Autodesk Fusion 360 part; units mm, degrees
(part 2 of 2)
  spline S382 degree 3 poles (93.789, 651.4002) (93.7155, 651.4002) (93.7155, 651.4737) (93.642, 651.4737) knots 0 0 0 0 1 1 1 1
  spline S383 degree 3 poles (93.642, 651.4737) (86.5858, 656.8394) (73.8699, 659.3385) (72.5468, 659.559) knots 0 0 0 0 1 1 1 1
  spline S384 degree 3 poles (72.5468, 659.559) (72.4733, 659.559) (72.3998, 659.559) (72.3263, 659.559) knots 0 0 0 0 1 1 1 1
  spline S385 degree 3 poles (72.3263, 659.559) (69.5332, 659.706) (66.7401, 659.7795) (63.947, 659.9265) knots 0 0 0 0 1 1 1 1
  spline S386 degree 3 poles (63.947, 659.9265) (63.5795, 659.9265) (63.212, 660) (62.8445, 660) knots 0 0 0 0 1 1 1 1
  spline S387 degree 3 poles (62.8445, 660) (62.6975, 660) (62.624, 660) (62.477, 660) knots 0 0 0 0 1 1 1 1
  spline S388 degree 3 poles (62.477, 660) (59.8309, 659.4855) (57.1848, 659.0445) (54.5387, 658.53) knots 0 0 0 0 1 1 1 1
  spline S389 degree 3 poles (54.5387, 658.53) (54.3917, 658.4565) (54.1712, 658.3829) (54.0242, 658.3094) knots 0 0 0 0 1 1 1 1
  spline S390 degree 3 poles (54.0242, 658.3094) (53.8772, 658.2359) (53.8037, 658.1624) (53.7302, 658.0889) knots 0 0 0 0 1 1 1 1
  line L13 (53.7302, 658.0889) -> (53.3627, 657.7214)
  spline S391 degree 3 poles (53.3627, 657.7214) (53.2892, 657.6479) (53.2157, 657.5744) (53.0687, 657.5009) knots 0 0 0 0 1 1 1 1
  spline S392 degree 3 poles (53.0687, 657.5009) (52.1867, 657.0599) (51.3781, 656.6924) (50.5696, 656.2514) knots 0 0 0 0 1 1 1 1
  line L14 (50.5696, 656.2514) -> (50.1286, 655.9574)
  spline S393 degree 3 poles (50.1286, 655.9574) (49.9816, 655.8104) (49.8346, 655.6634) (49.6876, 655.4429) knots 0 0 0 0 1 1 1 1
  spline S394 degree 3 poles (49.6876, 655.4429) (49.6141, 655.3694) (49.6141, 655.2223) (49.5406, 655.1488) knots 0 0 0 0 1 1 1 1
  spline S395 degree 3 poles (49.5406, 655.1488) (47.0415, 653.2378) (45.2039, 650.8857) (44.1014, 647.9456) knots 0 0 0 0 1 1 1 1
  spline S396 degree 3 poles (44.1014, 647.9456) (43.9544, 647.5781) (44.0279, 647.1371) (44.2484, 646.7696) knots 0 0 0 0 1 1 1 1
  spline S397 degree 3 poles (44.2484, 646.7696) (44.4689, 646.4021) (44.7629, 645.9611) (44.9834, 645.5935) knots 0 0 0 0 1 1 1 1
  spline S398 degree 3 poles (44.9834, 645.5935) (45.645, 644.7115) (46.3065, 643.8295) (47.0415, 642.874) knots 0 0 0 0 1 1 1 1
  spline S399 degree 3 poles (47.0415, 642.874) (51.6722, 636.1852) (56.2293, 629.3495) (60.9335, 622.7343) knots 0 0 0 0 1 1 1 1
  spline S400 degree 3 poles (60.9335, 622.7343) (62.2565, 620.8968) (62.5505, 618.9122) (62.918, 616.9276) knots 0 0 0 0 1 1 1 1
  spline S401 degree 3 poles (62.918, 616.9276) (63.4325, 613.6935) (63.8735, 610.4594) (64.3146, 607.2253) knots 0 0 0 0 1 1 1 1
  spline S402 degree 3 poles (64.3146, 607.2253) (64.4616, 606.1228) (64.2411, 605.0202) (63.653, 604.0647) knots 0 0 0 0 1 1 1 1
  spline S403 degree 3 poles (63.653, 604.0647) (62.771, 602.5212) (61.8155, 601.0511) (60.7864, 599.5811) knots 0 0 0 0 1 1 1 1
  spline S404 degree 3 poles (60.7864, 599.5811) (60.4189, 599.0666) (59.9044, 598.552) (59.3164, 598.258) knots 0 0 0 0 1 1 1 1
  spline S405 degree 3 poles (59.3164, 598.258) (57.4053, 597.376) (56.5233, 595.7589) (55.8618, 593.9214) knots 0 0 0 0 1 1 1 1
  spline S406 degree 3 poles (55.8618, 593.9214) (55.2738, 592.1573) (54.2447, 590.8343) (52.4072, 590.0258) knots 0 0 0 0 1 1 1 1
  spline S407 degree 3 poles (52.4072, 590.0258) (48.144, 588.0412) (43.8809, 585.9096) (39.6913, 583.7046) knots 0 0 0 0 1 1 1 1
  spline S408 degree 3 poles (39.6913, 583.7046) (36.6042, 582.014) (34.7666, 579.0004) (33.5906, 575.8398) knots 0 0 0 0 1 1 1 1
  spline S409 degree 3 poles (33.5906, 575.8398) (32.341, 572.4587) (31.8265, 568.8571) (30.6505, 565.476) knots 0 0 0 0 1 1 1 1
  spline S410 degree 3 poles (30.6505, 565.476) (30.577, 565.182) (30.43, 564.9615) (30.3565, 564.6674) knots 0 0 0 0 1 1 1 1
  spline S411 degree 3 poles (30.3565, 564.6674) (30.283, 564.4469) (30.283, 564.2999) (30.283, 564.0794) knots 0 0 0 0 1 1 1 1
  spline S412 degree 3 poles (30.283, 564.0794) (30.283, 563.6384) (30.3565, 563.1974) (30.3565, 562.6829) knots 0 0 0 0 1 1 1 1
  spline S413 degree 3 poles (30.3565, 562.6829) (30.3565, 560.3308) (29.9155, 558.1257) (29.0334, 556.1412) knots 0 0 0 0 1 1 1 1
  spline S414 degree 3 poles (29.0334, 556.1412) (28.9599, 556.0677) (28.9599, 555.9207) (28.9599, 555.8472) knots 0 0 0 0 1 1 1 1
  spline S415 degree 3 poles (28.9599, 555.8472) (28.6659, 554.0831) (28.3719, 552.6131) (28.2249, 551.0695) knots 0 0 0 0 1 1 1 1
  spline S416 degree 3 poles (28.2249, 551.0695) (27.7839, 547.6884) (27.6369, 544.3808) (29.842, 541.5142) knots 0 0 0 0 1 1 1 1
  spline S417 degree 3 poles (29.842, 541.5142) (31.2385, 539.6767) (33.0026, 538.1331) (34.3991, 536.3691) knots 0 0 0 0 1 1 1 1
  spline S418 degree 3 poles (34.3991, 536.3691) (34.9871, 535.634) (35.5016, 534.605) (35.4281, 533.723) knots 0 0 0 0 1 1 1 1
  spline S419 degree 3 poles (35.4281, 533.723) (35.3546, 531.8854) (35.2076, 530.1214) (34.9136, 528.2838) knots 0 0 0 0 1 1 1 1
  spline S420 degree 3 poles (34.9136, 528.2838) (34.7666, 527.1078) (33.2966, 526.6667) (32.5616, 527.4753) knots 0 0 0 0 1 1 1 1
  spline S421 degree 3 poles (32.5616, 527.4753) (32.1205, 527.9898) (31.606, 528.4308) (30.871, 528.6513) knots 0 0 0 0 1 1 1 1
  spline S422 degree 3 poles (30.871, 528.6513) (30.283, 528.8718) (29.6215, 528.6513) (29.3274, 528.1368) knots 0 0 0 0 1 1 1 1
  spline S423 degree 3 poles (29.3274, 528.1368) (28.6659, 527.1813) (28.2984, 526.0787) (28.0779, 524.9027) knots 0 0 0 0 1 1 1 1
  spline S424 degree 3 poles (28.0779, 524.9027) (27.8574, 523.9472) (26.6814, 523.5062) (25.8728, 524.0942) knots 0 0 0 0 1 1 1 1
  spline S425 degree 3 poles (25.8728, 524.0942) (25.3583, 524.5352) (24.7703, 524.9027) (24.1088, 525.1967) knots 0 0 0 0 1 1 1 1
  spline S426 degree 3 poles (24.1088, 525.1967) (23.3003, 525.5642) (21.9037, 525.7847) (21.0217, 525.5642) knots 0 0 0 0 1 1 1 1
  spline S427 degree 3 poles (21.0217, 525.5642) (16.0235, 524.3147) (12.0544, 521.4481) (8.3058, 518.067) knots 0 0 0 0 1 1 1 1
  spline S428 degree 3 poles (8.3058, 518.067) (7.7913, 517.626) (7.5708, 516.8174) (7.4972, 516.1559) knots 0 0 0 0 1 1 1 1
  spline S429 degree 3 poles (7.4972, 516.1559) (7.2032, 514.2448) (6.9092, 512.4073) (5.5127, 510.8637) knots 0 0 0 0 1 1 1 1
  spline S430 degree 3 poles (5.5127, 510.8637) (3.8956, 509.0997) (4.1161, 506.9681) (4.0426, 504.763) knots 0 0 0 0 1 1 1 1
  spline S431 degree 3 poles (4.0426, 504.763) (3.9691, 502.4845) (4.1161, 500.4999) (6.3212, 499.1769) knots 0 0 0 0 1 1 1 1
  spline S432 degree 3 poles (6.3212, 499.1769) (6.4682, 499.1034) (6.7622, 498.8094) (6.7622, 498.6623) knots 0 0 0 0 1 1 1 1
  spline S433 degree 3 poles (6.7622, 498.6623) (6.6152, 496.4573) (7.1297, 493.9582) (5.4392, 492.1941) knots 0 0 0 0 1 1 1 1
  spline S434 degree 3 poles (5.4392, 492.1941) (2.9401, 489.548) (1.6906, 486.6815) (1.9846, 483.0799) knots 0 0 0 0 1 1 1 1
  spline S435 degree 3 poles (1.9846, 483.0799) (2.2051, 480.8013) (1.9846, 478.5227) (2.0581, 476.2441) knots 0 0 0 0 1 1 1 1
  spline S436 degree 3 poles (2.0581, 476.2441) (2.0581, 475.3621) (2.7196, 474.1861) (3.4546, 473.598) knots 0 0 0 0 1 1 1 1
  spline S437 degree 3 poles (3.4546, 473.598) (5.5127, 472.0545) (6.0272, 469.6289) (5.9537, 467.4974) knots 0 0 0 0 1 1 1 1
  spline S438 degree 3 poles (5.9537, 467.4974) (5.7332, 462.4992) (4.1161, 457.7216) (2.4256, 452.9439) knots 0 0 0 0 1 1 1 1
  spline S439 degree 3 poles (2.4256, 452.9439) (1.2495, 449.5628) (1.1025, 445.8877) (0.294, 442.3596) knots 0 0 0 0 1 1 1 1
  spline S440 degree 3 poles (0.294, 442.3596) (-0.2205, 440.0075) (0.441, 437.8024) (1.6171, 436.2589) knots 0 0 0 0 1 1 1 1
  spline S441 degree 3 poles (1.6171, 436.2589) (3.3076, 434.1273) (5.6597, 432.2898) (8.5998, 431.9958) knots 0 0 0 0 1 1 1 1
  spline S442 degree 3 poles (8.5998, 431.9958) (9.1878, 431.9222) (9.8493, 432.5838) (10.3638, 433.0248) knots 0 0 0 0 1 1 1 1
  spline S443 degree 3 poles (10.3638, 433.0248) (11.8339, 434.3478) (12.7894, 434.1273) (13.3774, 432.2163) knots 0 0 0 0 1 1 1 1
  spline S444 degree 3 poles (13.3774, 432.2163) (14.48, 428.6881) (14.774, 425.0865) (13.9655, 421.4114) knots 0 0 0 0 1 1 1 1
  spline S445 degree 3 poles (13.9655, 421.4114) (13.6714, 420.0149) (13.7449, 418.4713) (13.5244, 417.0748) knots 0 0 0 0 1 1 1 1
  spline S446 degree 3 poles (13.5244, 417.0748) (13.4509, 416.3397) (13.0834, 415.6047) (12.8629, 414.8697) knots 0 0 0 0 1 1 1 1
  spline S447 degree 3 poles (12.8629, 414.8697) (12.7159, 414.7227) (12.6424, 414.5022) (12.4954, 414.3552) knots 0 0 0 0 1 1 1 1
  spline S448 degree 3 poles (12.4954, 414.3552) (11.3194, 410.533) (9.1143, 407.2989) (6.6887, 404.1383) knots 0 0 0 0 1 1 1 1
  spline S449 degree 3 poles (6.6887, 404.1383) (5.5862, 402.7418) (5.2922, 401.0512) (5.9537, 399.1402) knots 0 0 0 0 1 1 1 1
  spline S450 degree 3 poles (5.9537, 399.1402) (7.6443, 394.3625) (11.6869, 392.3045) (15.803, 390.3199) knots 0 0 0 0 1 1 1 1
  spline S451 degree 3 poles (15.803, 390.3199) (16.685, 389.8789) (17.5671, 389.6584) (18.4491, 389.2909) knots 0 0 0 0 1 1 1 1
  spline S452 degree 3 poles (18.4491, 389.2909) (20.1397, 388.5559) (22.0507, 388.8499) (22.7857, 390.4669) knots 0 0 0 0 1 1 1 1
  spline S453 degree 3 poles (22.7857, 390.4669) (24.6233, 394.5096) (28.3719, 396.4206) (31.3855, 399.1402) knots 0 0 0 0 1 1 1 1
  spline S454 degree 3 poles (31.3855, 399.1402) (32.8556, 400.5367) (34.3991, 401.8598) (35.7957, 403.3298) knots 0 0 0 0 1 1 1 1
  spline S455 degree 3 poles (35.7957, 403.3298) (37.4127, 405.0939) (38.9563, 403.5503) (40.4998, 403.4033) knots 0 0 0 0 1 1 1 1
  spline S456 degree 3 poles (40.4998, 403.4033) (41.6758, 403.3298) (41.4553, 402.2273) (41.6758, 401.4923) knots 0 0 0 0 1 1 1 1
  spline S457 degree 3 poles (41.6758, 401.4923) (43.0724, 397.5967) (40.7203, 394.4361) (39.5443, 391.1284) knots 0 0 0 0 1 1 1 1
  spline S458 degree 3 poles (39.5443, 391.1284) (39.5443, 391.0549) (39.5443, 391.0549) (39.4708, 390.9814) knots 0 0 0 0 1 1 1 1
  spline S459 degree 3 poles (39.4708, 390.9814) (38.9563, 390.0259) (38.5152, 388.9969) (38.0742, 387.9678) knots 0 0 0 0 1 1 1 1
  spline S460 degree 2 poles (38.0742, 387.9678) (38.0742, 387.8943) (38.0007, 387.8943) knots 0 0 0 1 1 1
  spline S461 degree 3 poles (38.0007, 387.8943) (37.6332, 387.1593) (37.1922, 386.4243) (36.8247, 385.6157) knots 0 0 0 0 1 1 1 1
  spline S462 degree 3 poles (36.8247, 385.6157) (36.8982, 385.6157) (37.0452, 385.6157) (37.1187, 385.6157) knots 0 0 0 0 1 1 1 1
  spline S463 degree 3 poles (37.1187, 385.6157) (35.5751, 381.5731) (34.3991, 377.604) (34.0316, 376.0604) knots 0 0 0 0 1 1 1 1
  spline S464 degree 3 poles (34.0316, 376.0604) (33.9581, 375.8399) (33.8846, 375.6194) (33.8111, 375.3254) knots 0 0 0 0 1 1 1 1
  spline S465 degree 3 poles (33.8111, 375.3254) (33.6641, 374.6639) (33.4436, 374.0024) (33.5171, 373.3408) knots 0 0 0 0 1 1 1 1
  spline S466 degree 3 poles (33.5171, 373.3408) (33.5906, 372.6793) (33.8111, 371.8708) (34.3256, 371.5768) knots 0 0 0 0 1 1 1 1
  spline S467 degree 3 poles (34.3256, 371.5768) (35.7957, 370.4743) (37.3392, 369.4452) (39.0298, 368.6367) knots 0 0 0 0 1 1 1 1
  spline S468 degree 3 poles (39.0298, 368.6367) (42.0434, 367.1667) (42.9254, 364.4471) (43.1459, 361.5805) knots 0 0 0 0 1 1 1 1
  spline S469 degree 3 poles (43.1459, 361.5805) (43.3664, 357.8318) (42.9989, 353.9362) (42.9989, 350.1876) knots 0 0 0 0 1 1 1 1
  spline S470 degree 3 poles (42.9989, 350.1876) (42.9989, 349.1586) (43.2929, 348.203) (43.2194, 347.174) knots 0 0 0 0 1 1 1 1
  spline S471 degree 3 poles (43.2194, 347.174) (43.0724, 342.9844) (42.8519, 338.8682) (42.4844, 334.6786) knots 0 0 0 0 1 1 1 1
  spline S472 degree 3 poles (42.4844, 334.6786) (42.4844, 334.2376) (41.6023, 333.5761) (41.0878, 333.4291) knots 0 0 0 0 1 1 1 1
  spline S473 degree 3 poles (41.0878, 333.4291) (40.1323, 333.2086) (39.0298, 333.282) (38.0742, 333.3556) knots 0 0 0 0 1 1 1 1
  spline S474 degree 3 poles (38.0742, 333.3556) (36.8982, 333.4291) (36.3102, 332.988) (35.9427, 331.959) knots 0 0 0 0 1 1 1 1
  spline S475 degree 3 poles (35.9427, 331.959) (34.0316, 326.7403) (33.5906, 321.4482) (35.7221, 316.156) knots 0 0 0 0 1 1 1 1
  spline S476 degree 3 poles (35.7221, 316.156) (35.9427, 315.6415) (35.9427, 314.98) (35.9427, 314.392) knots 0 0 0 0 1 1 1 1
  spline S477 degree 3 poles (35.9427, 314.392) (35.5751, 310.6433) (35.5751, 307.1152) (38.8092, 304.3221) knots 0 0 0 0 1 1 1 1
  spline S478 degree 3 poles (38.8092, 304.3221) (41.2348, 302.2641) (41.8963, 298.0009) (40.0588, 295.4283) knots 0 0 0 0 1 1 1 1
  spline S479 degree 3 poles (40.0588, 295.4283) (39.9118, 295.2078) (39.8383, 294.8403) (39.6178, 294.6933) knots 0 0 0 0 1 1 1 1
  spline S480 degree 3 poles (39.6178, 294.6933) (37.4862, 293.5173) (35.2811, 292.4147) (33.0761, 291.2387) knots 0 0 0 0 1 1 1 1
  spline S481 degree 3 poles (33.0761, 291.2387) (32.9291, 291.0917) (32.8556, 290.9447) (32.7086, 290.8712) knots 0 0 0 0 1 1 1 1
  spline S482 degree 3 poles (32.7086, 290.8712) (30.6505, 289.6216) (28.6659, 288.2251) (26.6079, 287.049) knots 0 0 0 0 1 1 1 1
  spline S483 degree 3 poles (26.6079, 287.049) (24.0353, 285.6525) (21.2422, 284.55) (18.5961, 283.374) knots 0 0 0 0 1 1 1 1
  line L15 (18.5961, 283.374) -> (17.9346, 282.8594)
  spline S484 degree 3 poles (17.9346, 282.8594) (16.097, 280.6544) (14.186, 278.3758) (12.3484, 276.1707) knots 0 0 0 0 1 1 1 1
  spline S485 degree 3 poles (12.3484, 276.1707) (12.1279, 275.8767) (11.8339, 275.5092) (11.4664, 275.4357) knots 0 0 0 0 1 1 1 1
  spline S486 degree 3 poles (11.4664, 275.4357) (8.9673, 274.4802) (8.8203, 272.3486) (8.5998, 270.07) knots 0 0 0 0 1 1 1 1
  spline S487 degree 3 poles (8.5998, 270.07) (8.3058, 267.2034) (8.0118, 264.1899) (7.2032, 261.4703) knots 0 0 0 0 1 1 1 1
  spline S488 degree 3 poles (7.2032, 261.4703) (6.5417, 259.1917) (5.0717, 257.1336) (4.0426, 255.0021) knots 0 0 0 0 1 1 1 1
  spline S489 degree 3 poles (4.0426, 255.0021) (3.6751, 254.267) (3.4546, 253.3115) (3.5281, 252.503) knots 0 0 0 0 1 1 1 1
  spline S490 degree 3 poles (3.5281, 252.503) (3.9691, 247.3578) (6.4682, 243.1682) (9.7758, 239.346) knots 0 0 0 0 1 1 1 1
  spline S491 degree 3 poles (9.7758, 239.346) (11.4664, 237.435) (12.8629, 235.3034) (14.627, 233.4658) knots 0 0 0 0 1 1 1 1
  spline S492 degree 3 poles (14.627, 233.4658) (19.9927, 227.9532) (23.1533, 220.897) (28.4454, 215.3843) knots 0 0 0 0 1 1 1 1
  spline S493 degree 3 poles (28.4454, 215.3843) (29.1069, 214.7227) (29.6215, 213.9142) (30.3565, 213.4732) knots 0 0 0 0 1 1 1 1
  spline S494 degree 3 poles (30.3565, 213.4732) (32.341, 212.1502) (32.9291, 210.1656) (33.2966, 208.034) knots 0 0 0 0 1 1 1 1
  spline S495 degree 3 poles (33.2966, 208.034) (34.0316, 203.5504) (35.3546, 199.2873) (37.6332, 195.3182) knots 0 0 0 0 1 1 1 1
  spline S496 degree 3 poles (37.6332, 195.3182) (40.4263, 190.32) (42.9254, 185.1013) (45.939, 180.2502) knots 0 0 0 0 1 1 1 1
  spline S497 degree 3 poles (45.939, 180.2502) (47.997, 176.9426) (50.6431, 174.076) (53.1422, 171.0624) knots 0 0 0 0 1 1 1 1
  spline S498 degree 3 poles (53.1422, 171.0624) (54.9063, 168.8573) (56.7438, 166.7257) (58.5079, 164.5207) knots 0 0 0 0 1 1 1 1
  spline S499 degree 3 poles (58.5079, 164.5207) (58.8754, 164.0061) (59.1694, 163.1976) (59.0224, 162.6831) knots 0 0 0 0 1 1 1 1
  spline S500 degree 3 poles (59.0224, 162.6831) (58.2139, 158.6405) (58.9489, 154.6713) (59.9044, 150.7757) knots 0 0 0 0 1 1 1 1
  spline S501 degree 3 poles (59.9044, 150.7757) (60.2719, 149.0852) (59.8309, 148.5706) (58.3609, 148.2766) knots 0 0 0 0 1 1 1 1
  spline S502 degree 3 poles (58.3609, 148.2766) (54.5388, 147.3946) (51.3047, 145.0425) (48.5116, 142.5434) knots 0 0 0 0 1 1 1 1
  spline S503 degree 3 poles (48.5116, 142.5434) (46.086, 140.3384) (44.1014, 137.3983) (43.0724, 133.9436) knots 0 0 0 0 1 1 1 1
  spline S504 degree 3 poles (43.0724, 133.9436) (42.1169, 130.489) (41.1613, 127.1079) (41.5288, 123.5063) knots 0 0 0 0 1 1 1 1
  line L16 (41.5288, 123.5063) -> (41.5288, 123.4328)
  spline S505 degree 3 poles (41.5288, 123.4328) (41.5288, 123.1388) (41.5288, 122.9183) (41.5288, 122.6243) knots 0 0 0 0 1 1 1 1
  spline S506 degree 3 poles (41.5288, 122.6243) (41.5288, 122.5508) (41.5288, 122.4038) (41.5288, 122.3303) knots 0 0 0 0 1 1 1 1
  spline S507 degree 3 poles (41.5288, 122.3303) (41.6758, 121.4482) (41.8228, 120.5662) (42.1169, 119.7577) knots 0 0 0 0 1 1 1 1
  spline S508 degree 3 poles (42.1169, 119.7577) (42.7049, 118.4347) (43.4399, 117.1116) (44.1014, 115.7886) knots 0 0 0 0 1 1 1 1
  spline S509 degree 3 poles (44.1014, 115.7886) (44.3219, 115.274) (44.8364, 114.9801) (45.4245, 115.0535) knots 0 0 0 0 1 1 1 1
  spline S510 degree 3 poles (45.4245, 115.0535) (46.674, 115.127) (47.9235, 115.2005) (49.1731, 115.2005) knots 0 0 0 0 1 1 1 1
  spline S511 degree 3 poles (49.1731, 115.2005) (49.9081, 115.2005) (50.6431, 115.0535) (51.3047, 114.7596) knots 0 0 0 0 1 1 1 1
  spline S512 degree 3 poles (51.3047, 114.7596) (56.8908, 112.334) (62.477, 109.8349) (67.4752, 106.3068) knots 0 0 0 0 1 1 1 1
  spline S513 degree 3 poles (67.4752, 106.3068) (67.6222, 106.1598) (67.7692, 106.0128) (67.9162, 105.7923) knots 0 0 0 0 1 1 1 1
  spline S514 degree 3 poles (67.9162, 105.7923) (68.0632, 105.7188) (68.2102, 105.7188) (68.3572, 105.6452) knots 0 0 0 0 1 1 1 1
  spline S515 degree 2 poles (68.3572, 105.6452) (72.3998, 102.1906) (69.6067, 95.9429) knots 0 0 0 1 1 1
  spline S516 degree 3 poles (69.6067, 95.9429) (68.7247, 94.1054) (67.9897, 92.0473) (66.8136, 90.3568) knots 0 0 0 0 1 1 1 1
  spline S517 degree 3 poles (66.8136, 90.3568) (64.3881, 86.9021) (63.506, 83.08) (63.1385, 78.9639) knots 0 0 0 0 1 1 1 1
  spline S518 degree 3 poles (63.1385, 78.9639) (63.065, 78.0084) (63.065, 76.9793) (62.6975, 76.1708) knots 0 0 0 0 1 1 1 1
  spline S519 degree 3 poles (62.6975, 76.1708) (61.154, 73.3042) (61.9625, 70.5847) (62.9915, 67.8651) knots 0 0 0 0 1 1 1 1
  spline S520 degree 3 poles (62.9915, 67.8651) (64.5351, 63.8224) (67.0341, 60.7353) (70.4153, 58.0893) knots 0 0 0 0 1 1 1 1
  spline S521 degree 3 poles (70.4153, 58.0893) (72.2528, 56.6927) (73.5024, 54.5612) (74.9724, 52.7236) knots 0 0 0 0 1 1 1 1
  spline S522 degree 3 poles (74.9724, 52.7236) (76.1484, 51.1801) (77.251, 49.6365) (78.28, 48.0194) knots 0 0 0 0 1 1 1 1
  spline S523 degree 3 poles (78.28, 48.0194) (78.3535, 47.8724) (78.427, 47.7254) (78.5005, 47.5784) knots 0 0 0 0 1 1 1 1
  line L17 (78.5005, 47.5784) -> (80.1911, 46.3289)
  spline S524 degree 3 poles (80.1911, 46.3289) (82.1756, 46.4024) (84.1602, 46.5494) (85.9243, 45.0793) knots 0 0 0 0 1 1 1 1
  spline S525 degree 3 poles (85.9243, 45.0793) (89.3054, 42.2863) (89.8934, 38.3171) (87.3943, 34.7155) knots 0 0 0 0 1 1 1 1
  spline S526 degree 3 poles (87.3943, 34.7155) (86.1448, 32.878) (84.7482, 31.0404) (83.5722, 29.2028) knots 0 0 0 0 1 1 1 1
  spline S527 degree 3 poles (83.5722, 29.2028) (83.0577, 28.3943) (82.8372, 27.4388) (82.4696, 26.6303) knots 0 0 0 0 1 1 1 1
  spline S528 degree 3 poles (82.4696, 26.6303) (82.4696, 26.4833) (82.4696, 26.3362) (82.4696, 26.1893) knots 0 0 0 0 1 1 1 1
  spline S529 degree 3 poles (82.4696, 26.1893) (82.3961, 22.3671) (82.4696, 18.4715) (82.2491, 14.6494) knots 0 0 0 0 1 1 1 1
  spline S530 degree 3 poles (82.2491, 14.6494) (82.1021, 12.7383) (81.3671, 10.8273) (80.9996, 8.9162) knots 0 0 0 0 1 1 1 1
  spline S531 degree 3 poles (80.9996, 8.9162) (80.8526, 8.3282) (80.7791, 7.5932) (81.0731, 7.1521) knots 0 0 0 0 1 1 1 1
  spline S532 degree 3 poles (81.0731, 7.1521) (82.4696, 4.7266) (83.9397, 2.301) (86.5123, 0.9044) knots 0 0 0 0 1 1 1 1
  spline S533 degree 3 poles (86.5123, 0.9044) (87.1003, 0.6104) (87.9088, 0.6104) (88.6438, 0.4634) knots 0 0 0 0 1 1 1 1
  spline S534 degree 3 poles (88.6438, 0.4634) (89.1584, 0.3164) (89.6729, 0.1694) (90.1139, 0.0225) knots 0 0 0 0 1 1 1 1
  spline S535 degree 3 poles (90.1139, 0.0225) (90.4079, -0.051) (90.7019, -0.051) (90.9959, 0.0225) knots 0 0 0 0 1 1 1 1
  spline S536 degree 3 poles (90.9959, 0.0225) (94.1565, 1.1985) (97.3906, 2.3745) (100.5512, 3.5506) knots 0 0 0 0 1 1 1 1
  spline S537 degree 3 poles (100.5512, 3.5506) (100.7717, 3.624) (100.9922, 3.9916) (101.1392, 4.2121) knots 0 0 0 0 1 1 1 1
  spline S538 degree 3 poles (101.1392, 4.2121) (101.4333, 4.6531) (101.5803, 5.4616) (101.9478, 5.5351) knots 0 0 0 0 1 1 1 1
  spline S539 degree 3 poles (101.9478, 5.5351) (103.7118, 5.9761) (105.5494, 6.2702) (107.3869, 6.4906) knots 0 0 0 0 1 1 1 1
  spline S540 degree 3 poles (107.3869, 6.4906) (108.122, 6.5641) (108.9305, 6.6377) (109.6655, 6.6377) knots 0 0 0 0 1 1 1 1
  spline S541 degree 3 poles (109.6655, 6.6377) (110.4005, 6.6377) (110.9886, 7.1522) (111.0621, 7.8137) knots 0 0 0 0 1 1 1 1
  spline S542 degree 3 poles (111.0621, 7.8137) (111.0621, 7.9607) (111.1356, 8.1077) (111.1356, 8.2547) knots 0 0 0 0 1 1 1 1
  spline S543 degree 3 poles (111.0621, 8.2547) (111.3561, 12.8853) (111.1356, 17.516) (114.2962, 21.2646) knots 0 0 0 0 1 1 1 1
  spline S544 degree 3 poles (114.2962, 21.2646) (114.6637, 21.7056) (115.3987, 21.9996) (115.9867, 22.2201) knots 0 0 0 0 1 1 1 1
  spline S545 degree 3 poles (115.9867, 22.2201) (121.5729, 24.2047) (127.1591, 26.4098) (131.7162, 30.2319) knots 0 0 0 0 1 1 1 1
  spline S546 degree 3 poles (131.7162, 30.2319) (133.9948, 32.1429) (135.5383, 34.9361) (137.5964, 37.1411) knots 0 0 0 0 1 1 1 1
  spline S547 degree 3 poles (137.5964, 37.1411) (140.022, 39.7872) (140.5365, 43.0213) (140.6835, 46.3289) knots 0 0 0 0 1 1 1 1
  spline S548 degree 3 poles (140.6835, 46.3289) (140.9775, 51.6946) (141.2715, 56.9868) (141.345, 62.3524) knots 0 0 0 0 1 1 1 1
  spline S549 degree 3 poles (141.345, 62.3524) (141.4185, 64.7045) (140.904, 67.0566) (140.757, 69.4086) knots 0 0 0 0 1 1 1 1
  spline S550 degree 3 poles (140.757, 69.4086) (140.61, 71.4667) (142.8886, 74.1863) (144.8731, 74.6273) knots 0 0 0 0 1 1 1 1
  spline S551 degree 3 poles (144.8731, 74.6273) (147.1517, 75.0683) (149.4303, 75.5093) (151.6353, 76.0973) knots 0 0 0 0 1 1 1 1
  spline S552 degree 3 poles (151.6353, 76.0973) (152.7379, 76.3914) (153.8404, 76.9058) (154.8694, 77.4939) knots 0 0 0 0 1 1 1 1
  spline S553 degree 3 poles (154.8694, 77.4939) (157.5155, 78.8905) (161.2641, 78.4494) (163.3957, 76.4648) knots 0 0 0 0 1 1 1 1
  spline S554 degree 3 poles (163.3957, 76.4648) (164.5718, 75.3623) (165.8948, 74.5538) (165.8948, 72.4222) knots 0 0 0 0 1 1 1 1
  spline S555 degree 3 poles (165.8948, 72.4222) (165.8948, 71.4667) (167.6588, 70.4376) (168.6879, 69.5556) knots 0 0 0 0 1 1 1 1
  spline S556 degree 3 poles (168.6879, 69.5556) (169.9374, 68.5266) (171.2605, 67.571) (172.51, 66.542) knots 0 0 0 0 1 1 1 1
  spline S557 degree 3 poles (172.51, 66.542) (173.245, 65.954) (173.7595, 65.072) (174.0536, 64.1899) knots 0 0 0 0 1 1 1 1
  spline S558 degree 3 poles (174.0536, 64.1899) (175.3031, 60.6618) (178.0227, 58.2363) (180.8893, 56.1047) knots 0 0 0 0 1 1 1 1
  spline S559 degree 3 poles (180.8893, 56.1047) (183.0944, 54.4876) (185.7404, 54.5612) (188.166, 55.6637) knots 0 0 0 0 1 1 1 1
  spline S560 degree 3 poles (188.166, 55.6637) (192.5761, 57.5747) (196.9128, 59.6328) (201.1759, 61.8379) knots 0 0 0 0 1 1 1 1
  spline S561 degree 3 poles (201.1759, 61.8379) (202.7195, 62.6464) (204.0425, 64.043) (205.4391, 65.1455) knots 0 0 0 0 1 1 1 1
  spline S562 degree 3 poles (205.4391, 65.1455) (206.3211, 65.8805) (207.2031, 66.7626) (208.0851, 67.4976) knots 0 0 0 0 1 1 1 1
  spline S563 degree 3 poles (208.0851, 67.4976) (209.9962, 69.1147) (210.9517, 72.7162) (209.6287, 74.7743) knots 0 0 0 0 1 1 1 1
  spline S564 degree 3 poles (209.6287, 74.7743) (207.5706, 77.9349) (208.8202, 81.2425) (208.7467, 84.4767) knots 0 0 0 0 1 1 1 1
  spline S565 degree 3 poles (208.7467, 84.4767) (208.7467, 85.0647) (208.4527, 85.7997) (208.0851, 86.3142) knots 0 0 0 0 1 1 1 1
  spline S566 degree 3 poles (208.0851, 86.3142) (206.7621, 88.1518) (204.6305, 88.5193) (202.7195, 89.4013) knots 0 0 0 0 1 1 1 1
  spline S567 degree 3 poles (202.7195, 89.4013) (199.4119, 90.9449) (196.5453, 93.3705) (194.1197, 96.3106) knots 0 0 0 0 1 1 1 1
  spline S568 degree 3 poles (194.1197, 96.3106) (190.0771, 101.1617) (187.578, 106.8949) (184.1969, 112.1871) knots 0 0 0 0 1 1 1 1
  spline S569 degree 3 poles (184.1969, 112.1871) (183.3884, 113.5101) (182.5063, 114.9067) (181.4038, 116.0092) knots 0 0 0 0 1 1 1 1
  spline S570 degree 3 poles (181.4038, 116.0092) (179.6397, 117.8467) (179.9337, 119.9048) (180.6688, 121.8894) knots 0 0 0 0 1 1 1 1
  spline S571 degree 3 poles (180.6688, 121.8894) (180.7423, 122.0364) (180.7423, 122.1099) (180.8158, 122.2569) knots 0 0 0 0 1 1 1 1
  spline S572 degree 3 poles (180.8158, 122.2569) (185.2994, 128.5781) (188.313, 133.2822) (189.7096, 135.4873) knots 0 0 0 0 1 1 1 1
  spline S573 degree 3 poles (189.7096, 135.4873) (190.0036, 135.8548) (190.2976, 136.2223) (190.5181, 136.8103) knots 0 0 0 0 1 1 1 1
  spline S574 degree 3 poles (190.5181, 136.8103) (192.9437, 142.5435) (194.3402, 148.5707) (195.0752, 154.7449) knots 0 0 0 0 1 1 1 1
  spline S575 degree 3 poles (195.0752, 154.7449) (195.6633, 159.5226) (197.9418, 163.3447) (200.7349, 167.0933) knots 0 0 0 0 1 1 1 1
  spline S576 degree 3 poles (200.7349, 167.0933) (202.94, 170.1069) (204.263, 173.5615) (203.822, 177.6777) knots 0 0 0 0 1 1 1 1
  spline S577 degree 3 poles (203.822, 177.6777) (202.94, 185.3219) (202.8665, 192.8927) (206.9826, 199.8019) knots 0 0 0 0 1 1 1 1
  spline S578 degree 3 poles (206.9826, 199.8019) (209.9227, 204.7265) (211.3193, 210.3127) (213.1568, 215.6784) knots 0 0 0 0 1 1 1 1
  spline S579 degree 3 poles (213.1568, 215.6784) (213.9654, 218.0304) (216.2439, 218.986) (217.7875, 220.6765) knots 0 0 0 0 1 1 1 1
  spline S580 degree 3 poles (217.7875, 220.6765) (217.9345, 220.8235) (218.8165, 220.3825) (219.1105, 220.0885) knots 0 0 0 0 1 1 1 1
  spline S581 degree 3 poles (219.1105, 220.0885) (220.5805, 218.6184) (221.2421, 216.7809) (221.6096, 214.8698) knots 0 0 0 0 1 1 1 1
  spline S582 degree 3 poles (221.6096, 214.8698) (221.7566, 213.9878) (222.0506, 212.5913) (222.6386, 212.3707) knots 0 0 0 0 1 1 1 1
  spline S583 degree 3 poles (222.6386, 212.3707) (224.1087, 211.7827) (225.7992, 211.5622) (227.3428, 211.6357) knots 0 0 0 0 1 1 1 1
  spline S584 degree 3 poles (227.3428, 211.6357) (228.4453, 211.6357) (229.5478, 212.3707) (230.6504, 212.8117) knots 0 0 0 0 1 1 1 1
  spline S585 degree 3 poles (230.6504, 212.8117) (231.0914, 212.9588) (231.7529, 213.1793) (231.8999, 213.6203) knots 0 0 0 0 1 1 1 1
  spline S586 degree 3 poles (231.8999, 213.6203) (232.2674, 214.3553) (232.7084, 214.9433) (233.2964, 215.3843) knots 0 0 0 0 1 1 1 1
  spline S587 degree 3 poles (233.2964, 215.3843) (234.252, 217.9569) (235.428, 221.191) (236.457, 223.7636) knots 0 0 0 0 1 1 1 1
  spline S588 degree 3 poles (236.457, 223.7636) (236.31, 225.1602) (236.163, 226.6302) (235.9425, 228.0267) knots 0 0 0 0 1 1 1 1
  spline S589 degree 3 poles (235.9425, 228.0267) (235.428, 231.5548) (234.399, 235.0095) (234.3255, 238.4641) knots 0 0 0 0 1 1 1 1
  spline S590 degree 3 poles (234.3255, 238.4641) (234.2519, 242.1392) (235.134, 245.8143) (235.575, 249.4894) knots 0 0 0 0 1 1 1 1
  spline S591 degree 3 poles (235.575, 249.4894) (236.163, 254.4876) (235.722, 259.3388) (233.2229, 263.8224) knots 0 0 0 0 1 1 1 1
  spline S592 degree 3 poles (233.2229, 263.8224) (232.5614, 265.0719) (231.6794, 266.248) (231.2383, 267.4975) knots 0 0 0 0 1 1 1 1
  spline S593 degree 3 poles (231.2383, 267.4975) (230.7973, 268.8941) (230.2828, 270.5111) (230.6503, 271.8342) knots 0 0 0 0 1 1 1 1
  spline S594 degree 3 poles (230.6503, 271.8342) (232.0469, 276.9793) (233.8844, 281.904) (236.898, 286.3141) knots 0 0 0 0 1 1 1 1
  spline S595 degree 3 poles (236.898, 286.3141) (238.0741, 288.0047) (237.5596, 289.9893) (235.7955, 291.0918) knots 0 0 0 0 1 1 1 1
  spline S596 degree 3 poles (235.7955, 291.0918) (234.105, 292.1208) (232.7084, 293.2969) (232.3409, 295.4284) knots 0 0 0 0 1 1 1 1
  spline S597 degree 3 poles (232.3409, 295.4284) (232.1939, 296.0899) (231.7529, 296.678) (231.6059, 297.3395) knots 0 0 0 0 1 1 1 1
  spline S598 degree 3 poles (231.6059, 297.3395) (230.8708, 300.2061) (230.6503, 303.0727) (232.4144, 305.7188) knots 0 0 0 0 1 1 1 1
  spline S599 degree 3 poles (232.4144, 305.7188) (233.8844, 307.8503) (235.0605, 309.6879) (236.016, 311.2314) knots 0 0 0 0 1 1 1 1
  spline S600 degree 3 poles (236.016, 311.2314) (236.31, 311.6724) (236.604, 312.187) (236.898, 312.628) knots 0 0 0 0 1 1 1 1
  spline S601 degree 3 poles (236.8245, 312.628) (239.6176, 317.4056) (240.2056, 319.4637) (240.2791, 320.4192) knots 0 0 0 0 1 1 1 1
  spline S602 degree 3 poles (240.2791, 320.4192) (240.2791, 320.7867) (240.4996, 321.1542) (240.8672, 321.3747) knots 0 0 0 0 1 1 1 1
  spline S603 degree 3 poles (240.8672, 321.3747) (241.0877, 321.5218) (241.2347, 321.6687) (241.2347, 321.8158) knots 0 0 0 0 1 1 1 1
  spline S604 degree 3 poles (241.2347, 321.8158) (241.4552, 322.6978) (241.6022, 323.7268) (241.6022, 324.6824) knots 0 0 0 0 1 1 1 1
  spline S605 degree 3 poles (241.6022, 324.6824) (241.8227, 327.1079) (241.0877, 327.9164) (238.8826, 328.8719) knots 0 0 0 0 1 1 1 1
  line L18 (111.0621, 8.2547) -> (111.1356, 8.2547)
  line L19 (236.8245, 312.628) -> (236.898, 312.628)
  dimension "d3" = 660
  constraint horizontal L6
  constraint horizontal L8
  constraint vertical L9
  constraint horizontal L10
  constraint vertical L11
  constraint coincident L8.start L11.end
  measures "d3" distance of L8.start L10.end
extrude "Extrude1" add sketch "Sketch1" along normal blind 20 contours S0 S1 S2 S3 S4 S5 S6 S7 S8 S9 S10 S11 S12 S13 S14 S15 S16 S17 S18 S19 S20 S21 S22 S23 S24 S25 S26 S27 S28 S29 S30 S31 S32 S33 S34 S35 S36 S37 S38 S39 S40 S41 S42 S43 S44 S45 S46 S47 S48 S49 S50 S51 L0 S52 S53 S54 S55 S56 S57 S58 S59 S60 S61 S62 S63 S64 S65 S66 S67 S68 S69 S70 S71 S72 S73 S74 S75 S76 S77 S78 S79 S80 S81 S82 S83 S84 S85 S86 S87 L1 S88 S89 L2 S90 S91 S92 S93 S94 S95 S96 S97 S98 S272 S273 S274 S275 S276 S277 S278 S279 S280 S281 S282 S283 S284 S285 S286 S287 S288 S289 S290 S291 S292 S293 S294 S295 S296 S297 S298 S299 S300 S301 S302 L6 S492 S493 S494 S495 S496 S497 S498 S499 S500 S501 S502 S503 S504 L16 S505 S506 S507 S508 S509 S510 S511 S512 S513 S514 S515 S516 S517 S518 S519 S520 | S0 S1 S2 S3 S4 S5 S6 S7 S8 S9 S10 S11 S12 S13 S14 S15 S16 S17 S18 S19 S20 S21 S22 S23 S24 S25 S26 S27 S28 S29 S30 S31 S32 S33 S34 S35 S36 S37 S38 S39 S40 S41 S42 S43 S44 S45 S46 S47 S48 S49 S50 S51 L0 S52 S53 S54 S55 S56 S57 S58 S59 S60 S61 S62 S63 S64 S65 S66 S67 S68 S69 S70 S71 S72 S73 S74 S75 S76 S77 S78 S79 S80 S81 S82 S83 S84 S85 S86 S87 L1 S88 S89 L2 S90 S91 S92 S93 S94 S95 S96 S97 S98 S272 S273 S274 S275 S276 S277 S278 S279 S280 S281 S282 S283 S284 S285 S286 S287 S288 S289 S290 S291 S292 S293 S294 S295 S296 S297 S298 S299 S300 S301 S302 L6 S303 S304 S305 S306 S307 S308 S309 S310 S311 S312 S313 S314 S315 S316 S317 S318 S319 S320 S321 S322 S323 S324 S325 S326 S327 S328 S329 S330 S331 S332 S333 S334 S335 S336 S337 S338 S339 S340 S341 S342 S343 S344 S345 S346 S347 S348 S349 S350 S351 S352 S353 S354 L12 S355 S356 S357 S358 S359 S360 S361 S362 S363 S364 S365 S366 S367 S368 S369 S370 S371 S372 S373 S374 S375 S376 S377 S378 S379 S380 S381 S382 S383 S384 S385 S386 S387 S388 S389 S390 L13 S391 S392 L14 S393 S394 S395 S396 S397 S398 S399 S400 S401 S402 S403 S404 S405 S406 S407 S408 S409 S410 S411 S412 S413 S414 S415 S416 S417 S418 S419 S420 S421 S422 S423 S424 S425 S426 S427 S428 S429 S430 S431 S432 S433 S434 S435 S436 S437 S438 S439 S440 S441 S442 S443 S444 S445 S446 S447 S448 S449 S450 S451 S452 S453 S454 S455 S456 S457 S458 S459 S460 S461 S462 S463 S464 S465 S466 S467 S468 S469 S470 S471 S472 S473 S474 S475 S476 S477 S478 S479 S480 S481 S482 S483 L15 S484 S485 S486 S487 S488 S489 S490 S491 S492 S520 S521 S522 S523 L17 S524 S525 S526 S527 S528 S529 S530 S531 S532 S533 S534 S535 S536 S537 S538 S539 S540 S541 S542 S543 S544 S545 S546 S547 S548 S549 S550 S551 S552 S553 S554 S555 S556 S557 S558 S559 S560 S561 S562 S563 S564 S565 S566 S567 S568 S569 S570 S571 S572 S573 S574 S575 S576 S577 S578 S579 S580 S581 S582 S583 S584 S585 S586 S587 S588 S589 S590 S591 S592 S593 S594 S595 S596 S597 S598 S599 S600 S601 S602 S603 S604 S605 L18 L19
